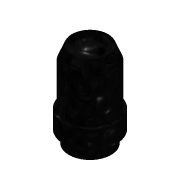
# Autodesk Inventor part: 30_CUBE_openSIM_ObjectiveLens_10x
Saved by Autodesk Inventor 2019 (Build 230136000, 136)
## iProperties
Created: 2019-10-21
Part Number: 30_CUBE_openSIM_ObjectiveLens_10x
Material: Generic
Document SubType Name: Modeling
Designer: diederichbenedict
Density: 1 g/cm^3
Appearance: Black
Author: diederichbenedict
Autodesk Inventor part; units mm, degrees
ref_plane "YZ Plane" through (0, 0, 0) normal (1, 0, 0) x (0, 1, 0)
ref_plane "XZ Plane" through (0, 0, 0) normal (0, 1, 0) x (-1, 0, 0)
ref_plane "XY Plane" through (0, 0, 0) normal (0, 0, 1) x (1, 0, 0)
sketch "Sketch1" plane through (0, 0, 0) normal (1, 0, 0) x (0, 1, 0)
  line L0 (0, 0) -> (0, -10.1)
  line L1 (0, -10.1) -> (5.8, -10.1)
  line L2 (5.8, -10.1) -> (5.8, -12.6)
  line L3 (5.8, -12.6) -> (14.4, -12.6)
  line L4 (14.4, -12.6) -> (14.4, -11.3)
  line L5 (14.4, -11.3) -> (34.4, -11.3)
  line L6 (34.4, -11.3) -> (40.8, -11.3)
  line L7 (40.8, -11.3) -> (40.8, -8.7)
  line L8 (40.8, -8.7) -> (34.4, -11.3)
  line L9 (40.8, -8.7) -> (43.8745, 0)
  line L10 (43.8745, 0) -> (0, 0)
  dimension "d0" = 10.1
  dimension "d1" = 5.8
  dimension "d2" = 90
  dimension "d3" = 2.5
  dimension "d4" = 90
  dimension "d5" = 8.6
  dimension "d6" = 1.3
  dimension "d7" = 90
  dimension "d8" = 20
  dimension "d9" = 6.4
  dimension "d10" = 2.6
  constraints: 22 end point, 7 perpendicular, 1 point on line, 1 vertical
  measures "d0" distance of L0.start L0.end
  measures "d1" distance of L0.end L1.end
  measures "d2" angle of L1 L0
  measures "d3" distance of L1.end L2.end
  measures "d4" angle of L1 L2
  measures "d5" distance of L2.end L3.end
  measures "d6" distance of L3.end L4.end
  measures "d7" angle of L4 L3
  measures "d8" distance of L4.end L5.end
  measures "d9" distance of L5.end L6.end
  measures "d10" distance of L6.end L7.end
revolve "Revolution1" add sketch "Sketch1" angle 360 about axis through (0, 43.8745, 0) along (0, -1, 0) contours L10 L9 L8 L5 L4 L3 L2 L1 L0
body "Solid1"
